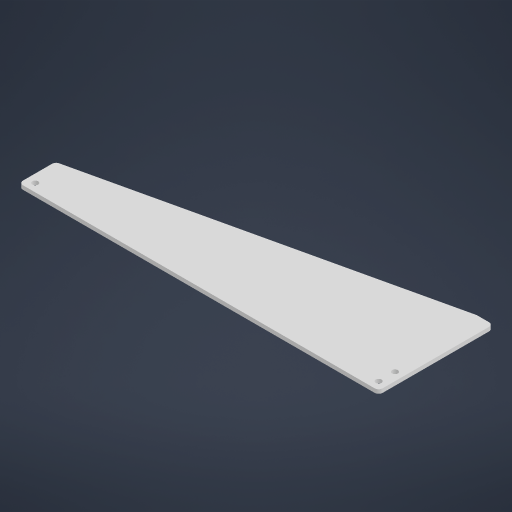
# Autodesk Inventor part: wing
Saved by Autodesk Inventor 2024 (Build 280153000, 153)
## iProperties
Created: 2023-08-30
Part Number: wing
Material: Generic
Document SubType Name: Sheet Metal
Designer: reima
Density: 1 g/cm^3
Sheet Metal Rule: Default
Appearance: Default
Author: reima
Autodesk Inventor part; units mm, degrees
ref_plane "YZ Plane" through (0, 0, 0) normal (1, 0, 0) x (0, 1, 0)
ref_plane "XZ Plane" through (0, 0, 0) normal (0, 1, 0) x (-1, 0, 0)
ref_plane "XY Plane" through (0, 0, 0) normal (0, 0, 1) x (1, 0, 0)
sketch "Sketch1" plane through (0, 0, 0) normal (0, 1, 0) x (-1, 0, 0)
  circle A0 centre (-4.2815, 25.8375) radius 2.2479
  circle A1 centre (-4.2815, 13.1375) radius 2.2479
  circle A2 centre (262.4185, 25.8375) radius 2.2479
  line L0 (-7.4565, 32.1875) -> (265.5935, 32.1875)
  line L1 (268.7685, 29.0125) -> (268.7685, 6.4355)
  line L2 (268.7489, 6.7875) -> (-10.6315, 6.7875)
  line L3 (-10.6315, 6.7875) -> (-10.6315, 29.0125)
  line L4 (-10.6315, 6.7875) -> (-10.6315, -53.5375)
  line L5 (-7.4565, -56.7125) -> (1.7122, -56.7125)
  line L6 (2.4159, -56.6335) -> (266.2971, 3.3395)
  arc A3 (1.7122, -56.7125) -> (2.4159, -56.6335) centre (1.7122, -53.5375) ccw
  arc A4 (-7.4565, 32.1875) -> (-10.6315, 29.0125) centre (-7.4565, 29.0125) ccw
  arc A5 (-10.6315, -53.5375) -> (-7.4565, -56.7125) centre (-7.4565, -53.5375) ccw
  arc A6 (266.2971, 3.3395) -> (268.7685, 6.4355) centre (265.5935, 6.4355) ccw
  arc A7 (268.7685, 29.0125) -> (265.5935, 32.1875) centre (265.5935, 29.0125) ccw
  point P0 (0, 0)
  point P1 (-10.6315, -56.7125)
  point P2 (2.0685, -56.7125)
  dimension "d0" = 4.4958
  dimension "d1" = 4.4958
  dimension "d2" = 12.7
  dimension "d3" = 4.4958
  dimension "d4" = 266.7
  dimension "d5" = 6.35
  dimension "d6" = 6.35
  dimension "d7" = 6.35
  dimension "d8" = 6.35
  dimension "d9" = 6.35
  dimension "d10" = 63.5
  dimension "d11" = 12.7
  dimension "d12" = 3.175
  measures "d0" diameter of A0
  measures "d1" diameter of A1
  measures "d2" distance of A1.centre A0.centre
  measures "d3" diameter of A2
  measures "d4" distance of A0.centre A2.centre
  measures "d5" distance from line of L1 A2.centre
  measures "d6" distance from line of L0 A2.centre
  measures "d7" distance from line of A0.centre L3
  measures "d8" distance from line of A1.centre L2
  measures "d9" distance from line of L0 A0.centre
  measures "d10" distance of L2.end point (-10.632, -56.712)
  measures "d11" distance of point (-10.632, -56.712) point (2.068, -56.712)
  measures "d12" radius of A3
extrude "Plate1" add sketch "Sketch1" along normal blind 3.048
equation "\"d13\" = Thickness"
equation "\"BendRadius\" = Thickness"
equation "\"BendReliefWidth\" = Thickness"
equation "\"BendReliefDepth\" = 0.5 * Thickness"
equation "\"CornerReliefSize\" = 4 * Thickness"
equation "\"MinimumRemnant\" = 2 * Thickness"
equation "\"TransitionRadius\" = BendRadius"
equation "\"JacobiRadiusSize\" = BendRadius"
equation "\"GapSize\" = Thickness"
equation "\"Thickness\" = 3.048"
body "Solid1"
